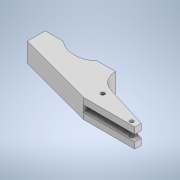
# Autodesk Inventor part: gripper3
Saved by Autodesk Inventor 2022 (Build 260153000, 153)
## iProperties
Created: 2022-01-15
Part Number: gripper3
Material: Generic
Document SubType Name: Modeling
Designer: nguye
Density: 1 g/cm^3
Appearance: Default
Author: nguye
Autodesk Inventor part; units mm, degrees
ref_plane "YZ Plane" through (0, 0, 0) normal (1, 0, 0) x (0, 1, 0)
ref_plane "XZ Plane" through (0, 0, 0) normal (0, 1, 0) x (-1, 0, 0)
ref_plane "XY Plane" through (0, 0, 0) normal (0, 0, 1) x (1, 0, 0)
sketch "Sketch1" plane through (0, 0, 0) normal (0, 1, 0) x (-1, 0, 0)
  line L0 (100, -16.077) -> (100, -30)
  line L1 (0, -5) -> (0, 0)
  line L2 (0, 0) -> (40, 0)
  line L3 (40, 0) -> (100, -16.077)
  line L4 (100, -16.077) -> (100, -26.077)
  line L5 (45, -30) -> (55, -30)
  arc A0 (45, -30) -> (34.4399, -15.6721) centre (30, -30) ccw
  line L6 (0, -5) -> (34.4399, -15.6721)
  arc A1 (85.7288, -30) -> (59.2712, -30) centre (72.5, -45) ccw
  line L7 (100, -30) -> (85.7288, -30)
  line L8 (59.2712, -30) -> (45, -30)
  constraints: 18 end point, 4 point on circle, 2 centre point, 2 point on line, 1 parallel, 1 tangent
extrude "Extrusion1" add sketch "Sketch1" along normal blind 15
sketch "Sketch2" plane through (0, 15, 0) normal (0, 1, 0) x (1, 0, 0)
  line L0 (0, 0) -> (0, 5) projected
  circle A0 centre (-5, 2.5) radius 1.5
  circle A1 centre (-35, 10) radius 1.5
  dimension "d14" = 3
  dimension "d17" = 3
  constraints: 2 centre point
  measures "d14" diameter of A0
  measures "d17" diameter of A1
extrude "Extrusion2" cut sketch "Sketch2" against normal blind 15
sketch "Sketch3" plane through (-40, 0, 0) normal (0, 0, 1) x (1, 0, 0)
  line L0 (40, 0) -> (40, 15) projected
  line L1 (40, 5) -> (0, 5)
  line L2 (0, 5) -> (0, 10)
  line L3 (0, 10) -> (40, 10)
  line L4 (40, 10) -> (40, 5)
  dimension "d20" = 5
  dimension "d21" = 40
  dimension "d22" = 5
  constraints: 8 end point, 2 parallel, 1 horizontal, 1 perpendicular, 1 point on line
  measures "d20" distance of L0.start L1.start
  measures "d21" distance of L2.end L3.end
  measures "d22" distance of L1.end L2.end
extrude "Extrusion3" cut sketch "Sketch3" against normal blind 44.75
body "Solid1"
